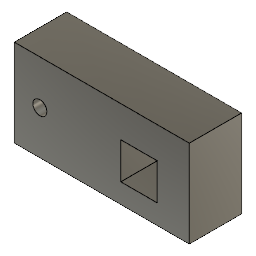
box (Autodesk Fusion 360 design; units mm, degrees)
Autodesk Fusion 360 part; units mm, degrees
box "BoxPrimitive1" add length 100 width 200 height 60 placed x (0, 0, 1) y (1, 0, 0) z (0, 1, 0) at (-155.2109, 0, -8.8747)
hole "Hole1" at (-125.851, 60, 40.8743) direction (0, -1, 0) diameter 16 depth 100 tip angle 118
sketch "Sketch7" plane through (0, 0, 0) normal (0, -1, 0) x (1, 0, 0)
  circle A0 centre (-125.851, 40.8743) radius 8
  line L0 (44.7891, 91.1253) -> (-155.2109, 91.1253)
  line L1 (-155.2109, 91.1253) -> (-155.2109, -8.8747)
  line L2 (-155.2109, -8.8747) -> (44.7891, -8.8747)
  line L3 (44.7891, -8.8747) -> (44.7891, 91.1253)
  line L4 (-33.4877, 55.3548) -> (8.1123, 55.3548)
  line L5 (8.1123, 55.3548) -> (8.1123, 13.7548)
  line L6 (8.1123, 13.7548) -> (-33.4877, 13.7548)
  line L7 (-33.4877, 13.7548) -> (-33.4877, 55.3548)
  dimension "d9" = 41.6
  dimension "d10" = 41.6
  measures "d9" distance of origin
  measures "d10" distance of origin
extrude "Extrude1" cut sketch "Sketch7" against normal blind 60 contours L4 L5 L6 L7
